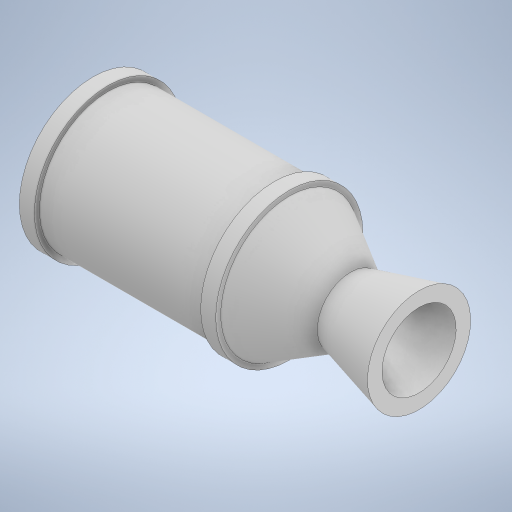
# Autodesk Inventor part: concept 2
Saved by Autodesk Inventor 2023 (Build 270158000, 158)
## iProperties
Created: 2022-09-14
Part Number: concept 2
Material: Generic
Document SubType Name: Modeling
Designer: station
Density: 1 g/cm^3
Appearance: Default
Author: station
Autodesk Inventor part; units mm, degrees
ref_plane "YZ Plane" through (0, 0, 0) normal (1, 0, 0) x (0, 1, 0)
ref_plane "XZ Plane" through (0, 0, 0) normal (0, 1, 0) x (-1, 0, 0)
ref_plane "XY Plane" through (0, 0, 0) normal (0, 0, 1) x (1, 0, 0)
sketch "Sketch1" plane through (0, 0, 0) normal (0, 0, 1) x (1, 0, 0)
  line L0 (0, 0) -> (0, 54.375) construction
  line L1 (0, 54.375) -> (192, 54.375)
  line L2 (0, 0) -> (524.135, 0)
  line L3 (254.7886, 18.124) -> (254.7886, 0) construction
  line L4 (192, 54.375) -> (254.7886, 18.124)
  line L5 (254.7886, 18.124) -> (325.1228, 36.97)
  line L6 (325.1228, 36.97) -> (325.1228, 0) construction
  line L7 (192, 54.375) -> (192, 0) construction
  line L8 (325.1228, 51.4639) -> (256.7665, 33.1479)
  line L9 (256.7665, 33.1479) -> (195.7513, 68.375)
  line L10 (195.7513, 68.375) -> (0, 68.375)
  line L11 (0, 54.375) -> (0, 68.375)
  line L12 (325.1228, 36.97) -> (325.1228, 51.4639)
  line L13 (0, 68.375) -> (0, 73.375)
  line L14 (0, 73.375) -> (15, 73.375)
  line L15 (15, 73.375) -> (15, 68.375)
  line L16 (195.7513, 68.375) -> (195.7513, 73.375)
  line L17 (195.7513, 73.375) -> (180.7513, 73.375)
  line L18 (180.7513, 73.375) -> (180.7513, 68.375)
  dimension "d0" = 54.375
  dimension "d1" = 192
  dimension "d2" = 18.124
  dimension "d3" = 30
  dimension "d4" = 15
  dimension "d5" = 36.97
  dimension "d6" = 14
  dimension "d8" = 5
  dimension "d9" = 15
  dimension "d10" = 5
  dimension "d11" = 15
  constraints: 38 end point, 7 perpendicular, 7 point on line, 4 vertical, 1 horizontal
  measures "d0" distance of L0.start L0.end
  measures "d1" distance of L0.end L1.end
  measures "d2" distance of L3.start L3.end
  measures "d3" angle of L2 L4
  measures "d4" angle of L2 L5
  measures "d5" distance of L5.end L6.end
  measures "d6" distance between parallel lines of L1 L10
  measures "d8" distance of L10.end L13.end
  measures "d9" distance of L13.end L14.end
  measures "d10" distance of L9.end L16.end
  measures "d11" distance of L16.end L17.end
revolve "Revolution1" add sketch "Sketch1" angle 360 about axis through (0, 0, 0) along (1, 0, 0)
sketch "Sketch2" plane through (0, 0, 0) normal (-1, 0, 0) x (0, 0, 1)
  point P0 (0, 0)
body "Solid1"
